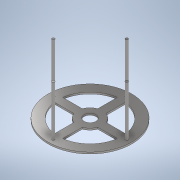
# Autodesk Inventor part: 8mm guide support
Saved by Autodesk Inventor 2020 (Build 240168000, 168)
## iProperties
Created: 2021-01-05
Part Number: 8mm guide support
Material: Steel, Mild
Document SubType Name: Modeling
Designer: Vikki
Density: 7.85 g/cm^3
Appearance: Semi-Polished
Author: Vikki
Autodesk Inventor part; units mm, degrees
ref_plane "YZ Plane" through (0, 0, 0) normal (1, 0, 0) x (0, 1, 0)
ref_plane "XZ Plane" through (0, 0, 0) normal (0, 1, 0) x (-1, 0, 0)
ref_plane "XY Plane" through (0, 0, 0) normal (0, 0, 1) x (1, 0, 0)
sketch "Sketch1" plane through (0, 0, 0) normal (0, 1, 0) x (-1, 0, 0)
  circle A0 centre (0, 0) radius 125
  circle A1 centre (110, 0) radius 4
  circle A2 centre (0, -110) radius 4
  circle A3 centre (-110, 0) radius 4
  circle A4 centre (0, 110) radius 4
  circle A5 centre (0, 0) radius 95
  dimension "d0" = 250
  dimension "d1" = 110
  dimension "d2" = 8
  dimension "d5" = 360
  dimension "d9" = 30
  constraints: 6 centre point, 2 coincident, 1 horizontal alignment, 9 other
  measures "d0" diameter of A0
  measures "d1" distance of point (0, 0) A1.centre
  measures "d2" diameter of A1
  measures "d9" radial gap between concentric circles of A0 A5
extrude "Extrusion1" add sketch "Sketch1" along normal blind 5
sketch "Sketch2" plane through (0, 5, 0) normal (0, 1, 0) x (1, 0, 0)
  circle A0 centre (0, 0) radius 125 projected
  circle A1 centre (-110, 0) radius 4 projected
  circle A2 centre (0, -110) radius 4 projected
  circle A3 centre (0, 0) radius 95 projected
  circle A4 centre (0, 110) radius 4 projected
  circle A5 centre (110, 0) radius 4 projected
extrude "Extrusion2" add sketch "Sketch2" along normal blind 150 and the other way blind 5 contours A1 | A2 | A4 | A5
sketch "Sketch3" plane through (0, 0, 0) normal (0, -1, 0) x (1, 0, 0)
  line L0 (-105, -12.5) -> (105, -12.5)
  line L1 (105, -12.5) -> (105, 12.5)
  line L2 (105, 12.5) -> (-105, 12.5)
  line L3 (-105, 12.5) -> (-105, -12.5)
  line L4 (-105, -12.5) -> (105, 12.5) construction
  line L5 (105, -12.5) -> (-105, 12.5) construction
  line L6 (-12.5, -105) -> (12.5, -105)
  line L7 (12.5, -105) -> (12.5, 105)
  line L8 (12.5, 105) -> (-12.5, 105)
  line L9 (-12.5, 105) -> (-12.5, -105)
  line L10 (-12.5, -105) -> (12.5, 105) construction
  line L11 (12.5, -105) -> (-12.5, 105) construction
  circle A0 centre (0, 0) radius 17.6
  circle A1 centre (0, 0) radius 37.6
  point P0 (35.4614, 12.5)
  point P1 (12.5, 35.4614)
  point P2 (-12.5, 35.4614)
  point P3 (-35.4614, 12.5)
  point P4 (-35.4614, -12.5)
  point P5 (-12.5, -35.4614)
  point P6 (12.5, -35.4614)
  point P7 (35.4614, -12.5)
  dimension "d14" = 210
  dimension "d15" = 25
  dimension "d16" = 35.2
  dimension "d17" = 20
  constraints: 24 end point, 4 midpoint, 4 parallel, 4 perpendicular, 2 centre point, 2 coincident, 2 horizontal
  measures "d14" distance of L0.start L0.end
  measures "d15" distance of L0.end L1.end
  measures "d16" diameter of A0
  measures "d17" radial gap between concentric circles of A0 A1
extrude "Extrusion3" add sketch "Sketch3" against normal blind 5 contours L3 L2 A1 L0 | A1 L2 L9 A0 L0 | L0 L9 A1 | L9 A0 L0 | L0 A0 L7 A1 L9 | A1 L9 L2 | A1 L7 L6 L9 | L9 A1 L7 L2 A0 | L2 A0 L9 | L9 L8 L7 A1 | L7 L0 A1 | A0 L7 L0 | A1 L2 L7 | L7 A0 L2 A1 L0 | A1 L2 L1 L0 | L2 L7 A0
body "Solid1"
